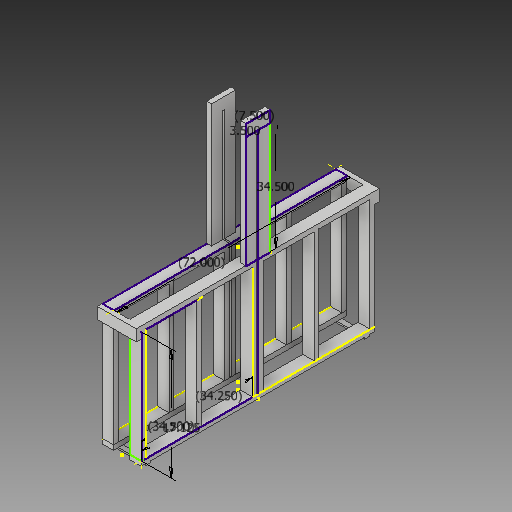
# Autodesk Inventor part: Trebuchet Base
Saved by Autodesk Inventor 2019 (Build 230136000, 136)
## iProperties
Created: 2019-07-10
Part Number: Trebuchet Base
Material: Generic
Document SubType Name: Modeling
Designer: AlphaGoldOmegaSilver
Density: 1 g/cm^3
Appearance: Default
Author: AlphaGoldOmegaSilver
Autodesk Inventor part; units mm, degrees
ref_plane "YZ Plane" through (0, 0, 0) normal (1, 0, 0) x (0, 1, 0)
ref_plane "XZ Plane" through (0, 0, 0) normal (0, 1, 0) x (-1, 0, 0)
ref_plane "XY Plane" through (0, 0, 0) normal (0, 0, 1) x (1, 0, 0)
sketch "Sketch1" plane through (0, 0, 0) normal (0, 1, 0) x (-1, 0, 0)
  line L0 (-152.4, 914.4) -> (152.4, 914.4) construction
  line L1 (152.4, 914.4) -> (152.4, -914.4) construction
  line L2 (152.4, -914.4) -> (-152.4, -914.4) construction
  line L3 (-152.4, -914.4) -> (-152.4, 914.4) construction
  line L4 (-152.4, 914.4) -> (152.4, -914.4) construction
  line L5 (152.4, 914.4) -> (-152.4, -914.4) construction
  line L6 (-152.4, 914.4) -> (-63.5, 914.4) construction
  line L7 (-63.5, 914.4) -> (-63.5, -914.4) construction
  line L8 (-63.5, -914.4) -> (-152.4, -914.4) construction
  line L9 (-152.4, -914.4) -> (-152.4, 914.4) construction
  line L10 (-152.4, 914.4) -> (-63.5, 914.4)
  line L11 (-63.5, 914.4) -> (-63.5, -914.4)
  line L12 (-63.5, -914.4) -> (-152.4, -914.4)
  line L13 (-152.4, -914.4) -> (-152.4, 914.4)
  line L14 (152.4, 914.4) -> (63.5, 914.4)
  line L15 (63.5, 914.4) -> (63.5, -914.4)
  line L16 (63.5, -914.4) -> (152.4, -914.4)
  line L17 (152.4, -914.4) -> (152.4, 914.4)
  point P0 (0, 0)
  dimension "d0" = 304.8
  dimension "d1" = 1828.8
  dimension "d2" = 88.9
  dimension "d3" = 88.9
  constraints: 36 end point, 8 parallel, 4 horizontal, 4 perpendicular, 2 midpoint, 2 point on line
  measures "d0" distance of L1.end L2.end
  measures "d1" distance of L0.end L1.end
  measures "d2" distance of L7.end L8.end
  measures "d3" distance of L16.end L15.end
extrude "Extrusion1" add sketch "Sketch1" along normal blind 38.1
sketch "Sketch2" plane through (0, 38.1, 0) normal (0, 1, 0) x (1, 0, 0)
  line L0 (-152.4, -914.4) -> (-63.5, -914.4) projected
  line L1 (-63.5, -914.4) -> (-63.5, 914.4) projected
  line L2 (-152.4, -914.4) -> (-63.5, -914.4)
  line L3 (-63.5, -914.4) -> (-63.5, -876.3)
  line L4 (-63.5, -876.3) -> (-152.4, -876.3)
  line L5 (-152.4, -876.3) -> (-152.4, -914.4)
  line L6 (63.5, -914.4) -> (152.4, -914.4) projected
  line L7 (152.4, -914.4) -> (63.5, -914.4)
  line L8 (63.5, -914.4) -> (63.5, -876.3)
  line L9 (63.5, -876.3) -> (152.4, -876.3)
  line L10 (152.4, -876.3) -> (152.4, -914.4)
  line L11 (-152.4, 914.4) -> (-152.4, -914.4) construction
  line L12 (152.4, -6.35) -> (-152.4, -6.35) construction
  line L13 (-152.4, -6.35) -> (-152.4, 6.35) construction
  line L14 (-152.4, 6.35) -> (152.4, 6.35) construction
  line L15 (152.4, 6.35) -> (152.4, -6.35) construction
  line L16 (152.4, -6.35) -> (-152.4, 6.35) construction
  line L17 (-152.4, -6.35) -> (152.4, 6.35) construction
  line L18 (-152.4, -6.35) -> (-63.5, -6.35)
  line L19 (-63.5, -6.35) -> (-63.5, -44.45)
  line L20 (-63.5, -44.45) -> (-152.4, -44.45)
  line L21 (-152.4, -44.45) -> (-152.4, -6.35)
  line L22 (-152.4, 6.35) -> (-63.5, 6.35)
  line L23 (-63.5, 6.35) -> (-63.5, 44.45)
  line L24 (-63.5, 44.45) -> (-152.4, 44.45)
  line L25 (-152.4, 44.45) -> (-152.4, 6.35)
  line L26 (152.4, 6.35) -> (63.5, 6.35)
  line L27 (63.5, 6.35) -> (63.5, 44.45)
  line L28 (63.5, 44.45) -> (152.4, 44.45)
  line L29 (152.4, 44.45) -> (152.4, 6.35)
  line L30 (152.4, -6.35) -> (63.5, -6.35)
  line L31 (63.5, -6.35) -> (63.5, -44.45)
  line L32 (63.5, -44.45) -> (152.4, -44.45)
  line L33 (152.4, -44.45) -> (152.4, -6.35)
  line L34 (107.95, -876.3) -> (107.95, -44.45) construction
  line L35 (-107.95, -876.3) -> (-107.95, -44.45) construction
  line L36 (153.186, -479.425) -> (62.714, -479.425)
  line L37 (62.714, -479.425) -> (62.714, -441.325)
  line L38 (62.714, -441.325) -> (153.186, -441.325)
  line L39 (153.186, -441.325) -> (153.186, -479.425)
  line L40 (153.186, -479.425) -> (62.714, -441.325) construction
  line L41 (62.714, -479.425) -> (153.186, -441.325) construction
  line L42 (-63.5, -479.425) -> (-152.4, -479.425)
  line L43 (-152.4, -479.425) -> (-152.4, -441.325)
  line L44 (-152.4, -441.325) -> (-63.5, -441.325)
  line L45 (-63.5, -441.325) -> (-63.5, -479.425)
  line L46 (-63.5, -479.425) -> (-152.4, -441.325) construction
  line L47 (-152.4, -479.425) -> (-63.5, -441.325) construction
  line L48 (152.4, 914.4) -> (63.5, 914.4) projected
  line L49 (152.4, -914.4) -> (152.4, 914.4) projected
  line L50 (63.5, 914.4) -> (152.4, 914.4)
  line L51 (152.4, 914.4) -> (152.4, 876.3)
  line L52 (152.4, 876.3) -> (63.5, 876.3)
  line L53 (63.5, 876.3) -> (63.5, 914.4)
  line L54 (-63.5, 914.4) -> (-152.4, 914.4) projected
  line L55 (-63.5, -914.4) -> (-63.5, 914.4) projected
  line L56 (-152.4, 914.4) -> (-63.5, 914.4)
  line L57 (-63.5, 914.4) -> (-63.5, 876.3)
  line L58 (-63.5, 876.3) -> (-152.4, 876.3)
  line L59 (-152.4, 876.3) -> (-152.4, 914.4)
  line L60 (-107.95, 44.45) -> (-107.95, 876.3) construction
  line L61 (107.95, 44.45) -> (107.95, 876.3) construction
  line L62 (-63.5, 441.325) -> (-152.4, 441.325)
  line L63 (-152.4, 441.325) -> (-152.4, 479.425)
  line L64 (-152.4, 479.425) -> (-63.5, 479.425)
  line L65 (-63.5, 479.425) -> (-63.5, 441.325)
  line L66 (-63.5, 441.325) -> (-152.4, 479.425) construction
  line L67 (-152.4, 441.325) -> (-63.5, 479.425) construction
  line L68 (63.5, 441.325) -> (152.4, 441.325)
  line L69 (152.4, 441.325) -> (152.4, 479.425)
  line L70 (152.4, 479.425) -> (63.5, 479.425)
  line L71 (63.5, 479.425) -> (63.5, 441.325)
  line L72 (63.5, 441.325) -> (152.4, 479.425) construction
  line L73 (152.4, 441.325) -> (63.5, 479.425) construction
  point P0 (0, 0)
  point P1 (107.95, -460.375)
  point P2 (-107.95, -460.375)
  point P3 (-107.95, 460.375)
  point P4 (107.95, 460.375)
  dimension "d6" = 38.1
  dimension "d8" = 12.7
  dimension "d9" = 38.1
  dimension "d10" = 38.1
  dimension "d11" = 38.1
  dimension "d17" = 38.1
  dimension "d18" = 38.1
  dimension "d19" = 88.9
  dimension "d20" = 38.1
  dimension "d21" = 88.9
  dimension "d22" = 38.1
  dimension "d23" = 38.1
  dimension "d24" = 88.9
  dimension "d25" = 88.9
  dimension "d26" = 88.9
  dimension "d27" = 38.1
  dimension "d28" = 38.1
  constraints: 132 end point, 26 parallel, 22 midpoint, 13 horizontal, 13 perpendicular, 9 point on line, 4 other
  measures "d6" distance of L3.end L2.end
  measures "d8" distance of L12.end L13.end
  measures "d9" distance of L18.end L19.end
  measures "d10" distance of L23.end L22.end
  measures "d11" distance of L36.end L37.end
  measures "d17" distance of L50.end L51.end
  measures "d18" distance of L56.end L57.end
  measures "d19" distance of L63.end L64.end
  measures "d20" distance of L62.end L63.end
  measures "d21" distance of L70.end L69.end
  measures "d22" distance of L69.end L68.end
  measures "d23" distance of L7.end L8.end
  measures "d24" distance of L6.end L7.end
  measures "d25" distance of L31.end L32.end
  measures "d26" distance of L27.end L28.end
  measures "d27" distance of L26.end L27.end
  measures "d28" distance of L30.end L31.end
extrude "Extrusion3" add sketch "Sketch2" along normal blind 876.3 separate body
sketch "Sketch10" plane through (0, 914.4, 0) normal (0, 1, 0) x (1, 0, 0)
  line L0 (-152.4, -914.4) -> (-63.5, -914.4) projected
  line L1 (-63.5, -6.35) -> (-152.4, -6.35) projected
  line L2 (-152.4, -914.4) -> (-63.5, -914.4)
  line L3 (-63.5, -914.4) -> (-63.5, -6.35)
  line L4 (-63.5, -6.35) -> (-152.4, -6.35)
  line L5 (-152.4, -6.35) -> (-152.4, -914.4)
  line L6 (152.4, -914.4) -> (152.4, -876.3) projected
  line L7 (63.5, -6.35) -> (152.4, -6.35)
  line L8 (152.4, -6.35) -> (152.4, -914.4)
  line L9 (152.4, -914.4) -> (63.5, -914.4)
  line L10 (63.5, -914.4) -> (63.5, -6.35)
  line L11 (-152.4, 6.35) -> (-63.5, 6.35) projected
  line L12 (-63.5, 914.4) -> (-152.4, 914.4) projected
  line L13 (-63.5, 6.35) -> (-152.4, 6.35)
  line L14 (-152.4, 6.35) -> (-152.4, 914.4)
  line L15 (-152.4, 914.4) -> (-63.5, 914.4)
  line L16 (-63.5, 914.4) -> (-63.5, 6.35)
  line L17 (63.5, 6.35) -> (152.4, 6.35) projected
  line L18 (63.5, 914.4) -> (152.4, 914.4)
  line L19 (152.4, 914.4) -> (152.4, 6.35)
  line L20 (152.4, 6.35) -> (63.5, 6.35)
  line L21 (63.5, 6.35) -> (63.5, 914.4)
  point P0 (0, 0)
  constraints: 32 end point, 8 parallel, 4 horizontal, 4 perpendicular
extrude "Extrusion7" add sketch "Sketch10" along normal blind 38.1 bodies 2
sketch "Sketch11" plane through (0, 952.5, 0) normal (0, 1, 0) x (1, 0, 0)
  line L0 (152.4, 6.35) -> (152.4, 914.4) projected
  line L1 (152.4, 6.35) -> (114.3, 6.35)
  line L2 (114.3, 6.35) -> (114.3, 95.25)
  line L3 (114.3, 95.25) -> (152.4, 95.25)
  line L4 (152.4, 95.25) -> (152.4, 6.35)
  line L5 (152.4, -6.35) -> (63.5, -6.35) projected
  line L6 (152.4, -6.35) -> (114.3, -6.35)
  line L7 (114.3, -6.35) -> (114.3, -95.25)
  line L8 (114.3, -95.25) -> (152.4, -95.25)
  line L9 (152.4, -95.25) -> (152.4, -6.35)
  line L10 (-152.4, 6.35) -> (-63.5, 6.35) projected
  line L11 (-152.4, 6.35) -> (-114.3, 6.35)
  line L12 (-114.3, 6.35) -> (-114.3, 95.25)
  line L13 (-114.3, 95.25) -> (-152.4, 95.25)
  line L14 (-152.4, 95.25) -> (-152.4, 6.35)
  line L15 (-152.4, -6.35) -> (-114.3, -6.35)
  line L16 (-114.3, -6.35) -> (-114.3, -95.25)
  line L17 (-114.3, -95.25) -> (-152.4, -95.25)
  line L18 (-152.4, -95.25) -> (-152.4, -6.35)
  point P0 (0, 0)
  dimension "d52" = 38.1
  dimension "d53" = 88.9
  dimension "d54" = 38.1
  dimension "d55" = 88.9
  dimension "d56" = 38.1
  dimension "d57" = 88.9
  dimension "d58" = 38.1
  dimension "d59" = 88.9
  constraints: 32 end point, 8 parallel, 4 horizontal, 4 perpendicular
  measures "d52" distance of L2.end L3.end
  measures "d53" distance of L1.end L2.end
  measures "d54" distance of L8.end L7.end
  measures "d55" distance of L7.end L6.end
  measures "d56" distance of L13.end L12.end
  measures "d57" distance of L12.end L11.end
  measures "d58" distance of L16.end L17.end
  measures "d59" distance of L15.end L16.end
extrude "Extrusion8" add sketch "Sketch11" along normal blind 876.3 bodies 2
sketch "Sketch13" plane through (0, 1828.8, 0) normal (0, 1, 0) x (1, 0, 0)
  line L0 (152.4, -95.25) -> (152.4, -6.35) projected
  line L1 (114.3, 95.25) -> (114.3, 6.35) projected
  line L2 (152.4, -95.25) -> (114.3, -95.25)
  line L3 (114.3, -95.25) -> (114.3, 95.25)
  line L4 (114.3, 95.25) -> (152.4, 95.25)
  line L5 (152.4, 95.25) -> (152.4, -95.25)
  line L6 (-152.4, 95.25) -> (-152.4, 6.35) projected
  line L7 (-152.4, 95.25) -> (-114.3, 95.25)
  line L8 (-114.3, 95.25) -> (-114.3, -95.25)
  line L9 (-114.3, -95.25) -> (-152.4, -95.25)
  line L10 (-152.4, -95.25) -> (-152.4, 95.25)
  point P0 (0, 0)
  constraints: 16 end point, 4 parallel, 2 horizontal, 2 perpendicular
extrude "Extrusion9" add sketch "Sketch13" along normal blind 88.9 bodies 2
sketch "Sketch16" plane through (0, 0, 0) normal (0, -1, 0) x (1, 0, 0)
  line L0 (-152.4, -876.3) -> (-63.5, -876.3) projected
  line L1 (152.4, 914.4) -> (152.4, -914.4) projected
  line L2 (-152.4, -876.3) -> (152.4, -876.3)
  line L3 (152.4, -876.3) -> (152.4, -838.2)
  line L4 (152.4, -838.2) -> (-152.4, -838.2)
  line L5 (-152.4, -838.2) -> (-152.4, -876.3)
  line L6 (-63.5, 876.3) -> (-152.4, 876.3) projected
  line L7 (-152.4, 876.3) -> (152.4, 876.3)
  line L8 (152.4, 876.3) -> (152.4, 838.2)
  line L9 (152.4, 838.2) -> (-152.4, 838.2)
  line L10 (-152.4, 838.2) -> (-152.4, 876.3)
  point P0 (0, 0)
  dimension "d75" = 38.1
  dimension "d76" = 38.1
  constraints: 16 end point, 4 parallel, 2 horizontal, 2 perpendicular, 2 point on line
  measures "d75" distance of L3.end L2.end
  measures "d76" distance of L7.end L8.end
extrude "Extrusion11" add sketch "Sketch16" along normal blind 12.7 bodies 1
sketch "Sketch17" plane through (-152.4, 38.1, 914.4) normal (0, 0, 1) x (1, 0, 0)
  line L0 (0, 914.4) -> (88.9, 914.4) projected
  line L1 (304.8, 0) -> (304.8, 914.4) projected
  line L2 (0, 914.4) -> (304.8, 914.4)
  line L3 (304.8, 914.4) -> (304.8, 825.5)
  line L4 (304.8, 825.5) -> (0, 825.5)
  line L5 (0, 825.5) -> (0, 914.4)
  point P0 (152.4, -38.1)
  dimension "d79" = 88.9
  constraints: 8 end point, 2 parallel, 1 horizontal, 1 perpendicular, 1 point on line
  measures "d79" distance of L2.end L3.end
extrude "Extrusion12" add sketch "Sketch17" along normal blind 38.1 bodies 2
sketch "Sketch18" plane through (-63.5, 38.1, -914.4) normal (0, 0, -1) x (-1, 0, 0)
  line L0 (88.9, 914.4) -> (88.9, 825.5) projected
  line L1 (-215.9, 825.5) -> (-127, 825.5) projected
  line L2 (88.9, 914.4) -> (-215.9, 914.4)
  line L3 (-215.9, 914.4) -> (-215.9, 825.5)
  line L4 (-215.9, 825.5) -> (88.9, 825.5)
  line L5 (88.9, 825.5) -> (88.9, 914.4)
  point P0 (-63.5, -38.1)
  constraints: 8 end point, 2 parallel, 1 horizontal, 1 perpendicular
extrude "Extrusion13" add sketch "Sketch18" along normal blind 38.1 bodies 2
sketch "Sketch19" plane through (152.4, 914.4, -44.45) normal (1, 0, 0) x (0, 0, -1)
  line L0 (-38.1, 914.4) -> (-50.8, 914.4) projected
  line L1 (-44.45, 914.4) -> (-44.45, -876.3)
  line L2 (-958.85, -876.3) -> (869.95, -876.3) projected
  point P0 (-44.45, -914.4)
  constraints: 2 end point, 2 midpoint
sketch "Sketch20" plane through (-152.4, 914.4, 44.45) normal (-1, 0, 0) x (0, 0, 1)
  line L0 (-50.8, 914.4) -> (-38.1, 914.4) projected
  line L1 (-44.45, 914.4) -> (-44.45, -876.3)
  line L2 (869.95, -876.3) -> (-958.85, -876.3) projected
  point P0 (-44.45, -914.4)
  constraints: 2 end point, 2 midpoint
sketch "Sketch21" plane through (152.4, 914.4, -44.45) normal (1, 0, 0) x (0, 0, -1)
  point P0 (-44.45, -914.4)
sketch "Sketch22" plane through (63.5, 38.1, 914.4) normal (0, 0, 1) x (1, 0, 0)
  line L0 (88.9, 0) -> (88.9, 876.3) projected
  line L1 (88.9, 876.3) -> (0, 876.3)
  line L2 (0, 876.3) -> (0, 0)
  line L3 (0, 0) -> (88.9, 0)
  line L4 (88.9, 0) -> (88.9, 876.3)
  point P0 (-63.5, -38.1)
  dimension "d84" = 876.3
  constraints: 8 end point, 2 parallel, 1 horizontal, 1 perpendicular
  measures "d84" distance of L0.start L0.end
sketch "Sketch23" plane through (0, 952.5, 0) normal (0, 1, 0) x (1, 0, 0)
  line L0 (-152.4, 914.4) -> (-63.5, 914.4)
  line L1 (-63.5, 914.4) -> (-63.5, -914.4)
  line L2 (-63.5, -914.4) -> (-152.4, -914.4)
  line L3 (-152.4, -914.4) -> (-152.4, 914.4)
  point P0 (0, 0)
  dimension "d85" = 1828.8
  constraints: 8 end point, 2 parallel, 1 horizontal, 1 perpendicular
  measures "d85" distance of L0.end L1.end
sketch "Sketch24" plane through (0, 38.1, 0) normal (0, 1, 0) x (1, 0, 0)
  point P0 (0, 0)
sketch "Sketch25" plane through (152.4, 914.4, -44.45) normal (1, 0, 0) x (0, 0, -1)
  point P0 (-44.45, -914.4)
sketch "Sketch26" plane through (152.4, 914.4, -44.45) normal (1, 0, 0) x (0, 0, -1)
  line L0 (-139.7, 38.1) -> (-139.7, 1003.3) projected
  line L1 (50.8, 914.4) -> (-139.7, 914.4)
  line L2 (-139.7, 914.4) -> (-139.7, 38.1)
  line L3 (-139.7, 38.1) -> (50.8, 38.1)
  line L4 (50.8, 38.1) -> (50.8, 914.4)
  point P0 (-44.45, -914.4)
  dimension "d87" = 876.3
  constraints: 8 end point, 2 parallel, 1 horizontal, 1 perpendicular
  measures "d87" distance of L3.end L1.start
sketch "Sketch27" plane through (152.4, 914.4, -44.45) normal (1, 0, 0) x (0, 0, -1)
  line L0 (50.8, 38.1) -> (50.8, 1003.3) projected
  line L1 (-139.7, 38.1) -> (-139.7, 1003.3) projected
  line L2 (50.8, 1003.3) -> (-139.7, 1003.3)
  line L3 (-139.7, 1003.3) -> (-139.7, 914.4)
  line L4 (-139.7, 914.4) -> (50.8, 914.4)
  line L5 (50.8, 914.4) -> (50.8, 1003.3)
  point P0 (-44.45, -914.4)
  dimension "d88" = 88.9
  dimension "d89" = 190.5
  constraints: 8 end point, 2 parallel, 1 horizontal, 1 perpendicular, 1 point on line
  measures "d88" distance of L3.end L2.end
  measures "d89" distance of L0.end L2.end
sketch "Sketch28" plane through (0, -12.7, 0) normal (0, -1, 0) x (1, 0, 0)
  point P0 (0, 0)
sketch "Sketch29" plane through (152.4, 0, -914.4) normal (1, 0, 0) x (0, 0, -1)
  line L0 (-1790.7, 38.1) -> (-1790.7, 914.4) projected
  line L1 (-1355.725, 914.4) -> (-1393.825, 914.4) projected
  line L2 (-1790.7, 914.4) -> (-1393.825, 914.4)
  line L3 (-1828.8, 38.1) -> (-1393.825, 38.1)
  line L4 (-1828.8, 38.1) -> (-1828.8, 863.6) projected
  line L5 (-958.85, 38.1) -> (-958.85, 914.4) projected
  line L6 (-1828.8, 38.1) -> (-958.85, 38.1)
  point P0 (-914.4, 0)
  dimension "d90" = 434.975
  dimension "d91" = 869.95
  constraints: 6 end point, 1 horizontal, 1 perpendicular
  measures "d90" distance of L3.start L3.end
  measures "d91" distance of L3.start L5.start
body "Solid1"
body "Solid2"
